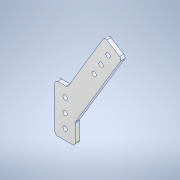
# Autodesk Inventor part: プレート保持_固定具3
Saved by Autodesk Inventor 2021 (Build 250183000, 183)
## iProperties
Created: 2022-02-09
Part Number: プレート保持_固定具3
Material: アルミニウム 6061
Document SubType Name: Modeling
Designer: hirohumi
Density: 2.7 g/cm^3
Appearance: アルミニウム - フラット
Author: hirohumi
Autodesk Inventor part; units mm, degrees
ref_plane "YZ Plane" through (0, 0, 0) normal (1, 0, 0) x (0, 1, 0)
ref_plane "XZ Plane" through (0, 0, 0) normal (0, 1, 0) x (-1, 0, 0)
ref_plane "XY Plane" through (0, 0, 0) normal (0, 0, 1) x (1, 0, 0)
sketch "スケッチ1" plane through (0, 0, 0) normal (0, 0, 1) x (1, 0, 0)
  line L0 (-157.5, 1000) -> (-142.5, 1000)
  line L1 (-142.5, 1000) -> (-142.5, 0) construction
  line L2 (-142.5, 0) -> (-157.5, 0) construction
  line L3 (-157.5, 0) -> (-157.5, 1000) construction
  line L4 (142.5, 500) -> (157.5, 500) construction
  line L5 (157.5, 500) -> (157.5, 0) construction
  line L6 (157.5, 0) -> (142.5, 0)
  line L7 (142.5, 0) -> (142.5, 500) construction
  circle A0 centre (-150, 0) radius 1.6
  circle A1 centre (150, 500) radius 1.6
  line L8 (127.3377, 476.8069) -> (140.2001, 469.0894) construction
  line L9 (140.2001, 469.0894) -> (-127.3377, 23.1931) construction
  line L10 (-127.3377, 23.1931) -> (-140.2001, 30.9106) construction
  line L11 (-140.2001, 30.9106) -> (127.3377, 476.8069) construction
  line L12 (-150, 0) -> (-133.7689, 27.0518) construction
  circle A2 centre (-150, 1000) radius 1.6
  circle A3 centre (150, 490) radius 1.6
  line L13 (133.7689, 472.9482) -> (150, 500) construction
  line L14 (-133.7689, 27.0518) -> (133.7689, 472.9482) construction
  circle A4 centre (128.6239, 464.3732) radius 1.6
  circle A5 centre (123.479, 455.7983) radius 1.6
  circle A6 centre (118.334, 447.2234) radius 1.6
  circle A7 centre (150, 510) radius 1.6
  circle A8 centre (128.6239, 535.6268) radius 1.6
  circle A9 centre (123.479, 544.2017) radius 1.6
  circle A10 centre (118.334, 552.7766) radius 1.6
  line L15 (157.5, 517.5) -> (157.5, 482.5)
  line L16 (157.5, 482.5) -> (148.2464, 482.5)
  line L17 (157.5, 517.5) -> (148.2464, 517.5)
  line L18 (148.2464, 517.5) -> (120.9065, 563.0665)
  line L19 (120.9065, 563.0665) -> (108.0441, 555.3491)
  line L20 (108.0441, 555.3491) -> (136.6231, 507.7174)
  line L21 (148.2464, 482.5) -> (120.9065, 436.9335)
  line L22 (120.9065, 436.9335) -> (108.0441, 444.6509)
  line L23 (108.0441, 444.6509) -> (136.6231, 492.2826)
  arc A11 (136.6231, 492.2826) -> (136.6231, 507.7174) centre (123.7607, 500) ccw
  line L24 (118.334, 552.7766) -> (128.6239, 535.6268) construction
  circle A12 centre (-150, 10) radius 1.6
  circle A13 centre (-128.6239, 35.6268) radius 1.6
  circle A14 centre (-123.479, 44.2017) radius 1.6
  circle A15 centre (-118.334, 52.7766) radius 1.6
  line L25 (-157.5, 17.5) -> (-148.2464, 17.5)
  line L26 (-148.2464, 17.5) -> (-120.9065, 63.0665)
  line L27 (-120.9065, 63.0665) -> (-108.0441, 55.3491)
  line L28 (-108.0441, 55.3491) -> (-142.5, -2.0774)
  line L29 (-142.5, -2.0774) -> (-142.5, -17.5)
  line L30 (-142.5, -17.5) -> (-157.5, -17.5)
  line L31 (-157.5, -17.5) -> (-157.5, 17.5)
  circle A16 centre (-150, -10) radius 1.6
  point P0 (0, 0)
  point P1 (0, 0)
  point P2 (150, 0)
  dimension "d0" = 15
  dimension "d1" = 15
  dimension "d2" = 1000
  dimension "d3" = 500
  dimension "d4" = 3.2
  dimension "d5" = 3.2
  dimension "d6" = 285
  dimension "d7" = 142.5
  dimension "d8" = 15
  dimension "d9" = 7.5
  dimension "d10" = 520
  dimension "d11" = 3.2
  dimension "d12" = 3.2
  dimension "d13" = 10
  dimension "d14" = 3.2
  dimension "d15" = 3.2
  dimension "d16" = 3.2
  dimension "d17" = 10
  dimension "d18" = 10
  dimension "d19" = 10
  dimension "d20" = 3.2
  dimension "d21" = 10
  dimension "d22" = 7.5
  dimension "d23" = 7.5
  dimension "d24" = 7.5
  dimension "d25" = 7.5
  dimension "d26" = 7.5
  dimension "d27" = 7.5
  dimension "d28" = 7.5
  dimension "d29" = 7.5
  dimension "d30" = 7.5
  dimension "d31" = 15
  dimension "d32" = 3.2
  dimension "d33" = 10
  dimension "d34" = 3.2
  dimension "d35" = 3.2
  dimension "d36" = 3.2
  dimension "d37" = 10
  dimension "d38" = 10
  dimension "d39" = 10
  dimension "d40" = 3.2
  dimension "d41" = 10
  dimension "d42" = 7.5
  dimension "d43" = 7.5
  dimension "d44" = 7.5
  dimension "d45" = 7.5
  dimension "d46" = 7.5
  constraints: 64 end point, 17 centre point, 12 parallel, 10 perpendicular, 9 point on line, 6 midpoint, 5 collinear, 4 vertical alignment, 3 horizontal, 3 symmetric about line, 2 horizontal alignment, 2 point on circle, 2 tangent, 1 coincident, 3 other
  measures "d0" distance of L1.end L2.end
  measures "d1" distance of L5.end L6.end
  measures "d2" distance of L2.end L0.start
  measures "d3" distance of L4.end L5.end
  measures "d4" diameter of A0
  measures "d5" diameter of A1
  measures "d6" distance between parallel lines of L7 L1
  measures "d7" distance from line of point (0, 0) L1
  measures "d8" distance of L8.start L8.end
  measures "d9" distance between parallel lines of L12 L11
  measures "d10" distance of L8.end L9.end
  measures "d11" diameter of A2
  measures "d12" diameter of A3
  measures "d13" distance of A3.centre L13.end
  measures "d14" diameter of A4
  measures "d15" diameter of A5
  measures "d16" diameter of A6
  measures "d17" distance of A5.centre A4.centre
  measures "d18" distance of A6.centre A5.centre
  measures "d19" distance from line of L8 A4.centre
  measures "d20" diameter of A7
  measures "d21" distance of A7.centre L13.end
  measures "d22" distance from line of L24.start L19
  measures "d23" distance between parallel lines of L18 L24
  measures "d24" distance between parallel lines of L24 L20
  measures "d25" distance between parallel lines of L21 L14
  measures "d26" distance between parallel lines of L14 L23
  measures "d27" distance from line of L22 A6.centre
  measures "d28" distance from line of A7.centre L15
  measures "d29" distance from line of L16 A3.centre
  measures "d30" distance from line of A7.centre L17
  measures "d31" radius of A11
  measures "d32" diameter of A12
  measures "d33" distance of L12.start A12.centre
  measures "d34" diameter of A13
  measures "d35" diameter of A14
  measures "d36" diameter of A15
  measures "d37" distance of A14.centre A13.centre
  measures "d38" distance of A15.centre A14.centre
  measures "d39" distance from line of L10 A13.centre
  measures "d40" diameter of A16
  measures "d41" distance of A16.centre L12.start
  measures "d42" distance from line of A15.centre L27
  measures "d43" distance between parallel lines of L14 L26
  measures "d44" distance from line of A12.centre L25
  measures "d45" distance from line of L30 A16.centre
  measures "d46" distance from line of L29 A16.centre
extrude "押し出し1" add sketch "スケッチ1" along normal blind 3 contours L25 L26 L27 L28 L29 L30 L31
fillet "フィレット1" radius 2 7 edges at (-120.9065, 63.0665, 1.5) (-108.0441, 55.3491, 1.5) (-142.5, -2.0774, 1.5) (-142.5, -17.5, 1.5) (-157.5, -17.5, 1.5) (-157.5, 17.5, 1.5) (-148.2464, 17.5, 1.5)
equation "\"d7\" = 0.5 * d6"
